Autodesk Fusion 360 part; units mm, degrees
(part 2 of 6)
  spline S50 degree 5 poles (26.1313, 46.3256) (26.12, 46.3173) (26.0976, 46.3005) (26.0639, 46.2753) (26.0191, 46.2416) (25.9633, 46.1993) (25.9077, 46.1569) (25.8522, 46.1143) (25.797, 46.0715) (25.7419, 46.0286) (25.687, 45.9856) (25.6324, 45.9424) (25.5779, 45.899) (25.5236, 45.8555) (25.4695, 45.8119) (25.4156, 45.768) (25.3619, 45.7241) (25.3084, 45.6799) (25.2552, 45.6356) (25.2021, 45.5912) (25.1492, 45.5466) (25.0966, 45.5018) (25.0441, 45.4569) (24.9919, 45.4118) (24.9399, 45.3665) (24.8881, 45.3211) (24.8365, 45.2755) (24.7851, 45.2297) (24.734, 45.1838) (24.6831, 45.1377) (24.6324, 45.0914) (24.582, 45.045) (24.5318, 44.9984) (24.4818, 44.9516) (24.4321, 44.9046) (24.3827, 44.8575) (24.3334, 44.8102) (24.2845, 44.7627) (24.2357, 44.7151) (24.1873, 44.6672) (24.1391, 44.6192) (24.0912, 44.571) (24.0435, 44.5226) (24.003, 44.481) (23.9721, 44.4491) (23.9507, 44.4268) (23.9388, 44.4144) (23.9362, 44.4117) knots -1 -1 -1 -1 -1 -1 -0.985714 -0.971429 -0.957143 -0.942857 -0.928571 -0.914286 -0.9 -0.885714 -0.871429 -0.857143 -0.842857 -0.828571 -0.814286 -0.8 -0.785714 -0.771429 -0.757143 -0.742857 -0.728571 -0.714286 -0.7 -0.685714 -0.671429 -0.657143 -0.642857 -0.628571 -0.614286 -0.6 -0.585714 -0.571429 -0.557143 -0.542857 -0.528571 -0.514286 -0.5 -0.485714 -0.471429 -0.457143 -0.442857 -0.428571 -0.414286 -0.4 -0.396066 -0.396066 -0.396066 -0.396066 -0.396066 -0.396066
  spline S51 degree 3 poles (23.3421, 44.3152) (23.3997, 44.2848) (23.4627, 44.266) (23.5923, 44.2536) (23.6577, 44.2602) (23.761, 44.2914) (23.8002, 44.309) (23.8731, 44.3538) (23.9066, 44.3808) (23.9362, 44.4117) knots 0 0 0 0 0.019532 0.019532 0.039064 0.039064 0.051902 0.051902 0.06474 0.06474 0.06474 0.06474
  arc A26 (23.3421, 44.3152) -> (22.9124, 44.5389) centre (0, 0) ccw
  spline S52 degree 3 poles (22.6507, 45.0809) (22.638, 45.017) (22.6379, 44.9513) (22.663, 44.8235) (22.6878, 44.7626) (22.7472, 44.6726) (22.7753, 44.64) (22.839, 44.5828) (22.8743, 44.5585) (22.9124, 44.5389) knots 0 0 0 0 0.019532 0.019532 0.039064 0.039064 0.051902 0.051902 0.06474 0.06474 0.06474 0.06474
  spline S53 degree 5 poles (22.6507, 45.0809) (22.6514, 45.0845) (22.6548, 45.1015) (22.6607, 45.1317) (22.6692, 45.1754) (22.68, 45.2324) (22.6923, 45.2992) (22.7043, 45.3661) (22.716, 45.4331) (22.7274, 45.5003) (22.7385, 45.5675) (22.7493, 45.6349) (22.7598, 45.7023) (22.77, 45.7699) (22.78, 45.8375) (22.7897, 45.9053) (22.799, 45.9731) (22.8081, 46.0411) (22.817, 46.1091) (22.8255, 46.1773) (22.8338, 46.2455) (22.8419, 46.3138) (22.8496, 46.3822) (22.8571, 46.4507) (22.8644, 46.5193) (22.8714, 46.5879) (22.8781, 46.6566) (22.8846, 46.7255) (22.8908, 46.7944) (22.8968, 46.8633) (22.9025, 46.9324) (22.908, 47.0015) (22.9132, 47.0707) (22.9182, 47.14) (22.9229, 47.2094) (22.9274, 47.2788) (22.9317, 47.3483) (22.9357, 47.4179) (22.9395, 47.4875) (22.9431, 47.5572) (22.9464, 47.627) (22.9495, 47.6968) (22.9523, 47.7667) (22.9549, 47.8367) (22.9569, 47.8927) (22.9582, 47.9347) (22.959, 47.9628) (22.9595, 47.9768) knots 0.396066 0.396066 0.396066 0.396066 0.396066 0.396066 0.4 0.414286 0.428571 0.442857 0.457143 0.471429 0.485714 0.5 0.514286 0.528571 0.542857 0.557143 0.571429 0.585714 0.6 0.614286 0.628571 0.642857 0.657143 0.671429 0.685714 0.7 0.714286 0.728571 0.742857 0.757143 0.771429 0.785714 0.8 0.814286 0.828571 0.842857 0.857143 0.871429 0.885714 0.9 0.914286 0.928571 0.942857 0.957143 0.971429 0.985714 1 1 1 1 1 1
  arc A27 (22.9595, 47.9768) -> (21.9943, 48.4269) centre (0, 0) ccw
  spline S54 degree 5 poles (21.9943, 48.4269) (21.9838, 48.4175) (21.9629, 48.3989) (21.9315, 48.3708) (21.8899, 48.3333) (21.8379, 48.2863) (21.7862, 48.2392) (21.7347, 48.192) (21.6834, 48.1446) (21.6323, 48.097) (21.5814, 48.0494) (21.5307, 48.0016) (21.4802, 47.9536) (21.4299, 47.9056) (21.3798, 47.8574) (21.33, 47.809) (21.2803, 47.7605) (21.2309, 47.7119) (21.1817, 47.6631) (21.1327, 47.6142) (21.0839, 47.5651) (21.0353, 47.5159) (20.987, 47.4666) (20.9389, 47.4171) (20.891, 47.3675) (20.8434, 47.3177) (20.796, 47.2678) (20.7488, 47.2178) (20.7019, 47.1676) (20.6552, 47.1172) (20.6087, 47.0667) (20.5625, 47.016) (20.5166, 46.9652) (20.4709, 46.9143) (20.4255, 46.8632) (20.3803, 46.8119) (20.3354, 46.7605) (20.2907, 46.7089) (20.2463, 46.6572) (20.2022, 46.6053) (20.1584, 46.5533) (20.1149, 46.501) (20.0716, 46.4487) (20.0349, 46.4038) (20.0069, 46.3692) (19.9875, 46.3452) (19.9767, 46.3318) (19.9744, 46.3288) knots -1 -1 -1 -1 -1 -1 -0.985714 -0.971429 -0.957143 -0.942857 -0.928571 -0.914286 -0.9 -0.885714 -0.871429 -0.857143 -0.842857 -0.828571 -0.814286 -0.8 -0.785714 -0.771429 -0.757143 -0.742857 -0.728571 -0.714286 -0.7 -0.685714 -0.671429 -0.657143 -0.642857 -0.628571 -0.614286 -0.6 -0.585714 -0.571429 -0.557143 -0.542857 -0.528571 -0.514286 -0.5 -0.485714 -0.471429 -0.457143 -0.442857 -0.428571 -0.414286 -0.4 -0.396066 -0.396066 -0.396066 -0.396066 -0.396066 -0.396066
  spline S55 degree 3 poles (19.391, 46.1809) (19.451, 46.1557) (19.5154, 46.1425) (19.6456, 46.1414) (19.7102, 46.1536) (19.8103, 46.1938) (19.8478, 46.2147) (19.9166, 46.2657) (19.9476, 46.2955) (19.9744, 46.3288) knots 0 0 0 0 0.019532 0.019532 0.039064 0.039064 0.051902 0.051902 0.06474 0.06474 0.06474 0.06474
  arc A28 (19.391, 46.1809) -> (18.9434, 46.3663) centre (0, 0) ccw
  spline S56 degree 3 poles (18.6354, 46.8834) (18.6284, 46.8187) (18.634, 46.7532) (18.6701, 46.6281) (18.7002, 46.5697) (18.7672, 46.4851) (18.798, 46.4551) (18.8664, 46.4037) (18.9038, 46.3825) (18.9434, 46.3663) knots 0 0 0 0 0.019532 0.019532 0.039064 0.039064 0.051902 0.051902 0.06474 0.06474 0.06474 0.06474
  spline S57 degree 5 poles (18.6354, 46.8834) (18.6358, 46.8872) (18.6377, 46.9043) (18.641, 46.935) (18.6456, 46.9792) (18.6514, 47.0369) (18.6578, 47.1046) (18.664, 47.1723) (18.6698, 47.2401) (18.6753, 47.3079) (18.6805, 47.3759) (18.6854, 47.4439) (18.69, 47.5121) (18.6943, 47.5802) (18.6983, 47.6485) (18.702, 47.7169) (18.7055, 47.7853) (18.7086, 47.8537) (18.7115, 47.9223) (18.7141, 47.9909) (18.7164, 48.0596) (18.7184, 48.1284) (18.7202, 48.1972) (18.7217, 48.2661) (18.723, 48.335) (18.7239, 48.404) (18.7246, 48.4731) (18.7251, 48.5422) (18.7253, 48.6114) (18.7252, 48.6806) (18.7249, 48.7499) (18.7243, 48.8192) (18.7235, 48.8886) (18.7224, 48.9581) (18.7211, 49.0276) (18.7196, 49.0971) (18.7177, 49.1667) (18.7157, 49.2364) (18.7134, 49.3061) (18.7109, 49.3758) (18.7081, 49.4456) (18.7051, 49.5155) (18.7018, 49.5854) (18.6984, 49.6553) (18.6954, 49.7113) (18.6931, 49.7533) (18.6914, 49.7813) (18.6906, 49.7953) knots 0.396066 0.396066 0.396066 0.396066 0.396066 0.396066 0.4 0.414286 0.428571 0.442857 0.457143 0.471429 0.485714 0.5 0.514286 0.528571 0.542857 0.557143 0.571429 0.585714 0.6 0.614286 0.628571 0.642857 0.657143 0.671429 0.685714 0.7 0.714286 0.728571 0.742857 0.757143 0.771429 0.785714 0.8 0.814286 0.828571 0.842857 0.857143 0.871429 0.885714 0.9 0.914286 0.928571 0.942857 0.957143 0.971429 0.985714 1 1 1 1 1 1
  arc A29 (18.6906, 49.7953) -> (17.6899, 50.1595) centre (0, 0) ccw
  spline S58 degree 5 poles (17.6899, 50.1595) (17.6803, 50.1493) (17.6611, 50.1289) (17.6323, 50.0982) (17.594, 50.0572) (17.5464, 50.0059) (17.499, 49.9544) (17.4518, 49.9029) (17.4048, 49.8512) (17.358, 49.7994) (17.3115, 49.7475) (17.2651, 49.6954) (17.219, 49.6433) (17.1731, 49.591) (17.1274, 49.5386) (17.082, 49.4861) (17.0367, 49.4335) (16.9917, 49.3807) (16.9469, 49.3278) (16.9024, 49.2748) (16.8581, 49.2217) (16.814, 49.1685) (16.7701, 49.1151) (16.7265, 49.0616) (16.6832, 49.008) (16.64, 48.9543) (16.5972, 48.9004) (16.5545, 48.8465) (16.5122, 48.7924) (16.47, 48.7381) (16.4282, 48.6838) (16.3866, 48.6293) (16.3452, 48.5747) (16.3041, 48.5199) (16.2633, 48.465) (16.2228, 48.41) (16.1825, 48.3549) (16.1426, 48.2996) (16.1029, 48.2442) (16.0634, 48.1887) (16.0243, 48.133) (15.9855, 48.0772) (15.947, 48.0213) (15.9143, 47.9733) (15.8894, 47.9365) (15.8722, 47.9109) (15.8626, 47.8965) (15.8605, 47.8934) knots -1 -1 -1 -1 -1 -1 -0.985714 -0.971429 -0.957143 -0.942857 -0.928571 -0.914286 -0.9 -0.885714 -0.871429 -0.857143 -0.842857 -0.828571 -0.814286 -0.8 -0.785714 -0.771429 -0.757143 -0.742857 -0.728571 -0.714286 -0.7 -0.685714 -0.671429 -0.657143 -0.642857 -0.628571 -0.614286 -0.6 -0.585714 -0.571429 -0.557143 -0.542857 -0.528571 -0.514286 -0.5 -0.485714 -0.471429 -0.457143 -0.442857 -0.428571 -0.414286 -0.4 -0.396066 -0.396066 -0.396066 -0.396066 -0.396066 -0.396066
  spline S59 degree 3 poles (15.2922, 47.6952) (15.3542, 47.6754) (15.4195, 47.6678) (15.5493, 47.6781) (15.6126, 47.6959) (15.7089, 47.7446) (15.7444, 47.7687) (15.8085, 47.8255) (15.8367, 47.8579) (15.8605, 47.8934) knots 0 0 0 0 0.019532 0.019532 0.039064 0.039064 0.051902 0.051902 0.06474 0.06474 0.06474 0.06474
  arc A30 (15.2922, 47.6952) -> (14.8302, 47.8409) centre (0, 0) ccw
  spline S60 degree 3 poles (14.4784, 48.3292) (14.477, 48.2641) (14.4883, 48.1994) (14.5351, 48.0779) (14.5702, 48.0223) (14.6443, 47.9439) (14.6776, 47.9167) (14.7502, 47.8715) (14.7893, 47.8536) (14.8302, 47.8409) knots 0 0 0 0 0.019532 0.019532 0.039064 0.039064 0.051902 0.051902 0.06474 0.06474 0.06474 0.06474
  spline S61 degree 5 poles (14.4784, 48.3292) (14.4784, 48.333) (14.4788, 48.3502) (14.4794, 48.3811) (14.4801, 48.4255) (14.4809, 48.4835) (14.4814, 48.5515) (14.4816, 48.6194) (14.4815, 48.6875) (14.4811, 48.7556) (14.4803, 48.8237) (14.4793, 48.8919) (14.4779, 48.9602) (14.4763, 49.0285) (14.4743, 49.0969) (14.4721, 49.1653) (14.4695, 49.2337) (14.4667, 49.3022) (14.4636, 49.3708) (14.4602, 49.4393) (14.4565, 49.508) (14.4525, 49.5766) (14.4483, 49.6453) (14.4438, 49.7141) (14.439, 49.7829) (14.434, 49.8517) (14.4287, 49.9206) (14.4231, 49.9895) (14.4173, 50.0584) (14.4112, 50.1274) (14.4048, 50.1964) (14.3982, 50.2654) (14.3913, 50.3345) (14.3842, 50.4035) (14.3768, 50.4727) (14.3692, 50.5418) (14.3614, 50.611) (14.3532, 50.6802) (14.3449, 50.7494) (14.3363, 50.8187) (14.3274, 50.888) (14.3183, 50.9573) (14.309, 51.0266) (14.2995, 51.096) (14.2916, 51.1515) (14.2856, 51.1931) (14.2816, 51.2209) (14.2796, 51.2348) knots 0.396066 0.396066 0.396066 0.396066 0.396066 0.396066 0.4 0.414286 0.428571 0.442857 0.457143 0.471429 0.485714 0.5 0.514286 0.528571 0.542857 0.557143 0.571429 0.585714 0.6 0.614286 0.628571 0.642857 0.657143 0.671429 0.685714 0.7 0.714286 0.728571 0.742857 0.757143 0.771429 0.785714 0.8 0.814286 0.828571 0.842857 0.857143 0.871429 0.885714 0.9 0.914286 0.928571 0.942857 0.957143 0.971429 0.985714 1 1 1 1 1 1
  arc A31 (14.2796, 51.2348) -> (13.2509, 51.5104) centre (0, 0) ccw
  spline S62 degree 5 poles (13.2509, 51.5104) (13.2422, 51.4994) (13.2248, 51.4774) (13.1988, 51.4443) (13.1643, 51.4002) (13.1213, 51.3449) (13.0786, 51.2895) (13.0361, 51.234) (12.9938, 51.1784) (12.9517, 51.1228) (12.9098, 51.067) (12.8682, 51.0111) (12.8268, 50.9551) (12.7856, 50.899) (12.7447, 50.8429) (12.704, 50.7866) (12.6635, 50.7302) (12.6232, 50.6737) (12.5832, 50.6172) (12.5435, 50.5605) (12.504, 50.5037) (12.4647, 50.4468) (12.4257, 50.3898) (12.3869, 50.3328) (12.3483, 50.2756) (12.3101, 50.2183) (12.272, 50.1609) (12.2343, 50.1034) (12.1968, 50.0458) (12.1596, 49.9881) (12.1226, 49.9303) (12.0859, 49.8724) (12.0495, 49.8144) (12.0133, 49.7563) (11.9774, 49.6981) (11.9419, 49.6397) (11.9065, 49.5813) (11.8715, 49.5228) (11.8368, 49.4641) (11.8024, 49.4053) (11.7683, 49.3465) (11.7345, 49.2875) (11.701, 49.2284) (11.6726, 49.1778) (11.651, 49.139) (11.6361, 49.1119) (11.6278, 49.0968) (11.626, 49.0935) knots -1 -1 -1 -1 -1 -1 -0.985714 -0.971429 -0.957143 -0.942857 -0.928571 -0.914286 -0.9 -0.885714 -0.871429 -0.857143 -0.842857 -0.828571 -0.814286 -0.8 -0.785714 -0.771429 -0.757143 -0.742857 -0.728571 -0.714286 -0.7 -0.685714 -0.671429 -0.657143 -0.642857 -0.628571 -0.614286 -0.6 -0.585714 -0.571429 -0.557143 -0.542857 -0.528571 -0.514286 -0.5 -0.485714 -0.471429 -0.457143 -0.442857 -0.428571 -0.414286 -0.4 -0.396066 -0.396066 -0.396066 -0.396066 -0.396066 -0.396066
  spline S63 degree 3 poles (11.0771, 48.8466) (11.1406, 48.8322) (11.2063, 48.8303) (11.3347, 48.8519) (11.3962, 48.8751) (11.4879, 48.932) (11.5212, 48.9592) (11.5801, 49.0213) (11.6054, 49.056) (11.626, 49.0935) knots 0 0 0 0 0.019532 0.019532 0.039064 0.039064 0.051902 0.051902 0.06474 0.06474 0.06474 0.06474
  arc A32 (11.0771, 48.8466) -> (10.6042, 48.9514) centre (0, 0) ccw
  spline S64 degree 3 poles (10.2111, 49.4072) (10.2154, 49.3422) (10.2323, 49.2787) (10.2896, 49.1618) (10.3293, 49.1094) (10.41, 49.0378) (10.4455, 49.0136) (10.5218, 48.9749) (10.5623, 48.9605) (10.6042, 48.9514) knots 0 0 0 0 0.019532 0.019532 0.039064 0.039064 0.051902 0.051902 0.06474 0.06474 0.06474 0.06474
  spline S65 degree 5 poles (10.2111, 49.4072) (10.2109, 49.4109) (10.2097, 49.4282) (10.2076, 49.4589) (10.2045, 49.5033) (10.2002, 49.5611) (10.1948, 49.6288) (10.189, 49.6966) (10.183, 49.7644) (10.1766, 49.8322) (10.17, 49.9) (10.163, 49.9678) (10.1557, 50.0357) (10.1481, 50.1036) (10.1402, 50.1715) (10.132, 50.2395) (10.1235, 50.3075) (10.1147, 50.3755) (10.1056, 50.4435) (10.0962, 50.5115) (10.0866, 50.5795) (10.0767, 50.6476) (10.0665, 50.7157) (10.056, 50.7838) (10.0452, 50.8519) (10.0342, 50.92) (10.0229, 50.9881) (10.0114, 51.0563) (9.9995, 51.1245) (9.9874, 51.1926) (9.9751, 51.2608) (9.9625, 51.329) (9.9496, 51.3972) (9.9365, 51.4654) (9.9232, 51.5336) (9.9095, 51.6019) (9.8957, 51.6701) (9.8816, 51.7383) (9.8672, 51.8066) (9.8526, 51.8748) (9.8377, 51.9431) (9.8226, 52.0113) (9.8073, 52.0796) (9.7917, 52.1478) (9.7791, 52.2025) (9.7695, 52.2434) (9.7631, 52.2707) (9.7598, 52.2844) knots 0.396066 0.396066 0.396066 0.396066 0.396066 0.396066 0.4 0.414286 0.428571 0.442857 0.457143 0.471429 0.485714 0.5 0.514286 0.528571 0.542857 0.557143 0.571429 0.585714 0.6 0.614286 0.628571 0.642857 0.657143 0.671429 0.685714 0.7 0.714286 0.728571 0.742857 0.757143 0.771429 0.785714 0.8 0.814286 0.828571 0.842857 0.857143 0.871429 0.885714 0.9 0.914286 0.928571 0.942857 0.957143 0.971429 0.985714 1 1 1 1 1 1
  arc A33 (9.7598, 52.2844) -> (8.7111, 52.4693) centre (0, 0) ccw
  spline S66 degree 5 poles (8.7111, 52.4693) (8.7034, 52.4576) (8.688, 52.4341) (8.665, 52.3989) (8.6344, 52.3519) (8.5964, 52.2931) (8.5587, 52.2342) (8.5211, 52.1752) (8.4838, 52.1162) (8.4468, 52.057) (8.4099, 51.9978) (8.3733, 51.9385) (8.337, 51.8791) (8.3008, 51.8197) (8.2649, 51.7602) (8.2293, 51.7006) (8.1939, 51.6409) (8.1587, 51.5811) (8.1238, 51.5212) (8.0891, 51.4613) (8.0547, 51.4013) (8.0205, 51.3412) (7.9866, 51.2811) (7.9529, 51.2208) (7.9196, 51.1605) (7.8864, 51.1001) (7.8535, 51.0396) (7.8209, 50.979) (7.7886, 50.9184) (7.7565, 50.8577) (7.7247, 50.7969) (7.6932, 50.736) (7.662, 50.675) (7.6311, 50.614) (7.6004, 50.5528) (7.57, 50.4916) (7.5399, 50.4303) (7.5102, 50.369) (7.4807, 50.3075) (7.4515, 50.246) (7.4227, 50.1844) (7.3941, 50.1227) (7.3659, 50.0609) (7.342, 50.008) (7.3239, 49.9674) (7.3114, 49.9392) (7.3045, 49.9234) (7.303, 49.92) knots -1 -1 -1 -1 -1 -1 -0.985714 -0.971429 -0.957143 -0.942857 -0.928571 -0.914286 -0.9 -0.885714 -0.871429 -0.857143 -0.842857 -0.828571 -0.814286 -0.8 -0.785714 -0.771429 -0.757143 -0.742857 -0.728571 -0.714286 -0.7 -0.685714 -0.671429 -0.657143 -0.642857 -0.628571 -0.614286 -0.6 -0.585714 -0.571429 -0.557143 -0.542857 -0.528571 -0.514286 -0.5 -0.485714 -0.471429 -0.457143 -0.442857 -0.428571 -0.414286 -0.4 -0.396066 -0.396066 -0.396066 -0.396066 -0.396066 -0.396066
  spline S67 degree 3 poles (6.7777, 49.6261) (6.8422, 49.6173) (6.9078, 49.6212) (7.0339, 49.6539) (7.0931, 49.6824) (7.1795, 49.7471) (7.2103, 49.777) (7.2635, 49.844) (7.2857, 49.8808) (7.303, 49.92) knots 0 0 0 0 0.019532 0.019532 0.039064 0.039064 0.051902 0.051902 0.06474 0.06474 0.06474 0.06474
  arc A34 (6.7777, 49.6261) -> (6.2974, 49.6893) centre (0, 0) ccw
  spline S68 degree 3 poles (5.8661, 50.1091) (5.876, 50.0448) (5.8984, 49.983) (5.9657, 49.8715) (6.0099, 49.8228) (6.0965, 49.7585) (6.134, 49.7375) (6.2134, 49.7055) (6.255, 49.6947) (6.2974, 49.6893) knots 0 0 0 0 0.019532 0.019532 0.039064 0.039064 0.051902 0.051902 0.06474 0.06474 0.06474 0.06474
  spline S69 degree 5 poles (5.8661, 50.1091) (5.8656, 50.1128) (5.8629, 50.1299) (5.8581, 50.1604) (5.8512, 50.2043) (5.8418, 50.2615) (5.8305, 50.3285) (5.8189, 50.3955) (5.807, 50.4625) (5.7947, 50.5295) (5.7822, 50.5965) (5.7693, 50.6635) (5.7561, 50.7304) (5.7426, 50.7974) (5.7288, 50.8644) (5.7147, 50.9314) (5.7003, 50.9984) (5.6857, 51.0653) (5.6707, 51.1323) (5.6554, 51.1992) (5.6399, 51.2662) (5.6241, 51.3331) (5.608, 51.4) (5.5916, 51.467) (5.575, 51.5339) (5.558, 51.6008) (5.5409, 51.6677) (5.5234, 51.7346) (5.5057, 51.8014) (5.4877, 51.8683) (5.4695, 51.9351) (5.451, 52.002) (5.4322, 52.0688) (5.4132, 52.1356) (5.3939, 52.2024) (5.3744, 52.2692) (5.3547, 52.3359) (5.3347, 52.4027) (5.3144, 52.4694) (5.2939, 52.5361) (5.2732, 52.6028) (5.2522, 52.6695) (5.231, 52.7362) (5.2095, 52.8028) (5.1921, 52.8561) (5.179, 52.8961) (5.1702, 52.9227) (5.1658, 52.936) knots 0.396066 0.396066 0.396066 0.396066 0.396066 0.396066 0.4 0.414286 0.428571 0.442857 0.457143 0.471429 0.485714 0.5 0.514286 0.528571 0.542857 0.557143 0.571429 0.585714 0.6 0.614286 0.628571 0.642857 0.657143 0.671429 0.685714 0.7 0.714286 0.728571 0.742857 0.757143 0.771429 0.785714 0.8 0.814286 0.828571 0.842857 0.857143 0.871429 0.885714 0.9 0.914286 0.928571 0.942857 0.957143 0.971429 0.985714 1 1 1 1 1 1
  arc A35 (5.1658, 52.936) -> (4.1049, 53.0289) centre (0, 0) ccw
  spline S70 degree 5 poles (4.1049, 53.0289) (4.0983, 53.0165) (4.085, 52.9918) (4.0651, 52.9547) (4.0388, 52.9052) (4.0061, 52.8433) (3.9736, 52.7814) (3.9413, 52.7193) (3.9093, 52.6573) (3.8776, 52.5951) (3.846, 52.5329) (3.8147, 52.4707) (3.7837, 52.4083) (3.7529, 52.346) (3.7223, 52.2835) (3.692, 52.221) (3.6619, 52.1585) (3.6321, 52.0959) (3.6025, 52.0332) (3.5732, 51.9705) (3.5441, 51.9077) (3.5153, 51.8449) (3.4868, 51.782) (3.4585, 51.719) (3.4305, 51.656) (3.4027, 51.593) (3.3753, 51.5299) (3.3481, 51.4667) (3.3211, 51.4035) (3.2945, 51.3402) (3.2681, 51.2768) (3.242, 51.2134) (3.2162, 51.15) (3.1907, 51.0865) (3.1655, 51.0229) (3.1406, 50.9593) (3.116, 50.8956) (3.0916, 50.8319) (3.0676, 50.7681) (3.0439, 50.7042) (3.0206, 50.6403) (2.9975, 50.5764) (2.9748, 50.5124) (2.9556, 50.4576) (2.9411, 50.4156) (2.9311, 50.3864) (2.9256, 50.37) (2.9244, 50.3665) knots -1 -1 -1 -1 -1 -1 -0.985714 -0.971429 -0.957143 -0.942857 -0.928571 -0.914286 -0.9 -0.885714 -0.871429 -0.857143 -0.842857 -0.828571 -0.814286 -0.8 -0.785714 -0.771429 -0.757143 -0.742857 -0.728571 -0.714286 -0.7 -0.685714 -0.671429 -0.657143 -0.642857 -0.628571 -0.614286 -0.6 -0.585714 -0.571429 -0.557143 -0.542857 -0.528571 -0.514286 -0.5 -0.485714 -0.471429 -0.457143 -0.442857 -0.428571 -0.414286 -0.4 -0.396066 -0.396066 -0.396066 -0.396066 -0.396066 -0.396066
  spline S71 degree 3 poles (2.4267, 50.028) (2.4918, 50.0248) (2.5568, 50.0344) (2.6795, 50.078) (2.736, 50.1115) (2.8164, 50.1835) (2.8445, 50.216) (2.8917, 50.2874) (2.9106, 50.326) (2.9244, 50.3665) knots 0 0 0 0 0.019532 0.019532 0.039064 0.039064 0.051902 0.051902 0.06474 0.06474 0.06474 0.06474
  arc A36 (2.4267, 50.028) -> (1.9427, 50.0491) centre (0, 0) ccw
  spline S72 degree 3 poles (1.4765, 50.4297) (1.492, 50.3665) (1.5197, 50.3069) (1.5964, 50.2017) (1.6446, 50.157) (1.7365, 50.1005) (1.7757, 50.0828) (1.8576, 50.0579) (1.9, 50.0508) (1.9427, 50.0491) knots 0 0 0 0 0.019532 0.019532 0.039064 0.039064 0.051902 0.051902 0.06474 0.06474 0.06474 0.06474
  spline S73 degree 5 poles (1.4765, 50.4297) (1.4756, 50.4334) (1.4715, 50.4501) (1.4641, 50.4801) (1.4533, 50.5232) (1.439, 50.5794) (1.4219, 50.6452) (1.4045, 50.7109) (1.3868, 50.7766) (1.3688, 50.8423) (1.3504, 50.9079) (1.3317, 50.9735) (1.3128, 51.0391) (1.2935, 51.1046) (1.2739, 51.1702) (1.254, 51.2356) (1.2339, 51.3011) (1.2134, 51.3665) (1.1926, 51.4319) (1.1716, 51.4973) (1.1503, 51.5626) (1.1287, 51.6279) (1.1068, 51.6932) (1.0847, 51.7585) (1.0623, 51.8237) (1.0396, 51.8888) (1.0166, 51.954) (0.9934, 52.0191) (0.9699, 52.0842) (0.9462, 52.1492) (0.9222, 52.2142) (0.898, 52.2792) (0.8734, 52.3441) (0.8487, 52.409) (0.8237, 52.4739) (0.7984, 52.5387) (0.7729, 52.6035) (0.7472, 52.6682) (0.7212, 52.7329) (0.6949, 52.7976) (0.6685, 52.8622) (0.6417, 52.9268) (0.6148, 52.9914) (0.5876, 53.0559) (0.5657, 53.1075) (0.5491, 53.1462) (0.538, 53.1719) (0.5325, 53.1848) knots 0.396066 0.396066 0.396066 0.396066 0.396066 0.396066 0.4 0.414286 0.428571 0.442857 0.457143 0.471429 0.485714 0.5 0.514286 0.528571 0.542857 0.557143 0.571429 0.585714 0.6 0.614286 0.628571 0.642857 0.657143 0.671429 0.685714 0.7 0.714286 0.728571 0.742857 0.757143 0.771429 0.785714 0.8 0.814286 0.828571 0.842857 0.857143 0.871429 0.885714 0.9 0.914286 0.928571 0.942857 0.957143 0.971429 0.985714 1 1 1 1 1 1
  arc A37 (0.5325, 53.1848) -> (-0.5325, 53.1848) centre (0, 0) ccw
  spline S74 degree 5 poles (-0.5325, 53.1848) (-0.538, 53.1719) (-0.5491, 53.1462) (-0.5657, 53.1075) (-0.5876, 53.0559) (-0.6148, 52.9914) (-0.6417, 52.9268) (-0.6685, 52.8622) (-0.6949, 52.7976) (-0.7212, 52.7329) (-0.7472, 52.6682) (-0.7729, 52.6035) (-0.7984, 52.5387) (-0.8237, 52.4739) (-0.8487, 52.409) (-0.8734, 52.3441) (-0.898, 52.2792) (-0.9222, 52.2142) (-0.9462, 52.1492) (-0.9699, 52.0842) (-0.9934, 52.0191) (-1.0166, 51.954) (-1.0396, 51.8888) (-1.0623, 51.8237) (-1.0847, 51.7585) (-1.1068, 51.6932) (-1.1287, 51.6279) (-1.1503, 51.5626) (-1.1716, 51.4973) (-1.1926, 51.4319) (-1.2134, 51.3665) (-1.2339, 51.3011) (-1.254, 51.2356) (-1.2739, 51.1702) (-1.2935, 51.1046) (-1.3128, 51.0391) (-1.3317, 50.9735) (-1.3504, 50.9079) (-1.3688, 50.8423) (-1.3868, 50.7766) (-1.4045, 50.7109) (-1.4219, 50.6452) (-1.439, 50.5794) (-1.4533, 50.5232) (-1.4641, 50.4801) (-1.4715, 50.4501) (-1.4756, 50.4334) (-1.4765, 50.4297) knots -1 -1 -1 -1 -1 -1 -0.985714 -0.971429 -0.957143 -0.942857 -0.928571 -0.914286 -0.9 -0.885714 -0.871429 -0.857143 -0.842857 -0.828571 -0.814286 -0.8 -0.785714 -0.771429 -0.757143 -0.742857 -0.728571 -0.714286 -0.7 -0.685714 -0.671429 -0.657143 -0.642857 -0.628571 -0.614286 -0.6 -0.585714 -0.571429 -0.557143 -0.542857 -0.528571 -0.514286 -0.5 -0.485714 -0.471429 -0.457143 -0.442857 -0.428571 -0.414286 -0.4 -0.396066 -0.396066 -0.396066 -0.396066 -0.396066 -0.396066
  spline S75 degree 3 poles (-1.9427, 50.0491) (-1.8777, 50.0516) (-1.8137, 50.0669) (-1.6953, 50.1209) (-1.6419, 50.1593) (-1.5681, 50.238) (-1.543, 50.2728) (-1.5022, 50.3481) (-1.4867, 50.3882) (-1.4765, 50.4297) knots 0 0 0 0 0.019532 0.019532 0.039064 0.039064 0.051902 0.051902 0.06474 0.06474 0.06474 0.06474
  arc A38 (-1.9427, 50.0491) -> (-2.4267, 50.028) centre (0, 0) ccw
  spline S76 degree 3 poles (-2.9244, 50.3665) (-2.9034, 50.3049) (-2.8706, 50.2479) (-2.785, 50.1498) (-2.7331, 50.1095) (-2.6366, 50.0612) (-2.596, 50.047) (-2.5123, 50.0293) (-2.4695, 50.0259) (-2.4267, 50.028) knots 0 0 0 0 0.019532 0.019532 0.039064 0.039064 0.051902 0.051902 0.06474 0.06474 0.06474 0.06474
  spline S77 degree 5 poles (-2.9244, 50.3665) (-2.9256, 50.37) (-2.9311, 50.3864) (-2.9411, 50.4156) (-2.9556, 50.4576) (-2.9748, 50.5124) (-2.9975, 50.5764) (-3.0206, 50.6403) (-3.0439, 50.7042) (-3.0676, 50.7681) (-3.0916, 50.8319) (-3.116, 50.8956) (-3.1406, 50.9593) (-3.1655, 51.0229) (-3.1907, 51.0865) (-3.2162, 51.15) (-3.242, 51.2134) (-3.2681, 51.2768) (-3.2945, 51.3402) (-3.3211, 51.4035) (-3.3481, 51.4667) (-3.3753, 51.5299) (-3.4027, 51.593) (-3.4305, 51.656) (-3.4585, 51.719) (-3.4868, 51.782) (-3.5153, 51.8449) (-3.5441, 51.9077) (-3.5732, 51.9705) (-3.6025, 52.0332) (-3.6321, 52.0959) (-3.6619, 52.1585) (-3.692, 52.221) (-3.7223, 52.2835) (-3.7529, 52.346) (-3.7837, 52.4083) (-3.8147, 52.4707) (-3.846, 52.5329) (-3.8776, 52.5951) (-3.9093, 52.6573) (-3.9413, 52.7193) (-3.9736, 52.7814) (-4.0061, 52.8433) (-4.0388, 52.9052) (-4.0651, 52.9547) (-4.085, 52.9918) (-4.0983, 53.0165) (-4.1049, 53.0289) knots 0.396066 0.396066 0.396066 0.396066 0.396066 0.396066 0.4 0.414286 0.428571 0.442857 0.457143 0.471429 0.485714 0.5 0.514286 0.528571 0.542857 0.557143 0.571429 0.585714 0.6 0.614286 0.628571 0.642857 0.657143 0.671429 0.685714 0.7 0.714286 0.728571 0.742857 0.757143 0.771429 0.785714 0.8 0.814286 0.828571 0.842857 0.857143 0.871429 0.885714 0.9 0.914286 0.928571 0.942857 0.957143 0.971429 0.985714 1 1 1 1 1 1
  arc A39 (-4.1049, 53.0289) -> (-5.1658, 52.936) centre (0, 0) ccw
  spline S78 degree 5 poles (-5.1658, 52.936) (-5.1702, 52.9227) (-5.179, 52.8961) (-5.1921, 52.8561) (-5.2095, 52.8028) (-5.231, 52.7362) (-5.2522, 52.6695) (-5.2732, 52.6028) (-5.2939, 52.5361) (-5.3144, 52.4694) (-5.3347, 52.4027) (-5.3547, 52.3359) (-5.3744, 52.2692) (-5.3939, 52.2024) (-5.4132, 52.1356) (-5.4322, 52.0688) (-5.451, 52.002) (-5.4695, 51.9351) (-5.4877, 51.8683) (-5.5057, 51.8014) (-5.5234, 51.7346) (-5.5409, 51.6677) (-5.558, 51.6008) (-5.575, 51.5339) (-5.5916, 51.467) (-5.608, 51.4) (-5.6241, 51.3331) (-5.6399, 51.2662) (-5.6554, 51.1992) (-5.6707, 51.1323) (-5.6857, 51.0653) (-5.7003, 50.9984) (-5.7147, 50.9314) (-5.7288, 50.8644) (-5.7426, 50.7974) (-5.7561, 50.7304) (-5.7693, 50.6635) (-5.7822, 50.5965) (-5.7947, 50.5295) (-5.807, 50.4625) (-5.8189, 50.3955) (-5.8305, 50.3285) (-5.8418, 50.2615) (-5.8512, 50.2043) (-5.8581, 50.1604) (-5.8629, 50.1299) (-5.8656, 50.1128) (-5.8661, 50.1091) knots -1 -1 -1 -1 -1 -1 -0.985714 -0.971429 -0.957143 -0.942857 -0.928571 -0.914286 -0.9 -0.885714 -0.871429 -0.857143 -0.842857 -0.828571 -0.814286 -0.8 -0.785714 -0.771429 -0.757143 -0.742857 -0.728571 -0.714286 -0.7 -0.685714 -0.671429 -0.657143 -0.642857 -0.628571 -0.614286 -0.6 -0.585714 -0.571429 -0.557143 -0.542857 -0.528571 -0.514286 -0.5 -0.485714 -0.471429 -0.457143 -0.442857 -0.428571 -0.414286 -0.4 -0.396066 -0.396066 -0.396066 -0.396066 -0.396066 -0.396066
  spline S79 degree 3 poles (-6.2974, 49.6893) (-6.2328, 49.6975) (-6.1704, 49.7183) (-6.0571, 49.7824) (-6.0073, 49.8253) (-5.9407, 49.9102) (-5.9186, 49.9471) (-5.8846, 50.0256) (-5.8726, 50.0668) (-5.8661, 50.1091) knots 0 0 0 0 0.019532 0.019532 0.039064 0.039064 0.051902 0.051902 0.06474 0.06474 0.06474 0.06474
  arc A40 (-6.2974, 49.6893) -> (-6.7777, 49.6261) centre (0, 0) ccw
  spline S80 degree 3 poles (-7.303, 49.92) (-7.2767, 49.8604) (-7.2391, 49.8065) (-7.1453, 49.7162) (-7.09, 49.6806) (-6.9897, 49.6409) (-6.9481, 49.6303) (-6.8631, 49.62) (-6.8201, 49.6203) (-6.7777, 49.6261) knots 0 0 0 0 0.019532 0.019532 0.039064 0.039064 0.051902 0.051902 0.06474 0.06474 0.06474 0.06474
  spline S81 degree 5 poles (-7.303, 49.92) (-7.3045, 49.9234) (-7.3114, 49.9392) (-7.3239, 49.9674) (-7.342, 50.008) (-7.3659, 50.0609) (-7.3941, 50.1227) (-7.4227, 50.1844) (-7.4515, 50.246) (-7.4807, 50.3075) (-7.5102, 50.369) (-7.5399, 50.4303) (-7.57, 50.4916) (-7.6004, 50.5528) (-7.6311, 50.614) (-7.662, 50.675) (-7.6932, 50.736) (-7.7247, 50.7969) (-7.7565, 50.8577) (-7.7886, 50.9184) (-7.8209, 50.979) (-7.8535, 51.0396) (-7.8864, 51.1001) (-7.9196, 51.1605) (-7.9529, 51.2208) (-7.9866, 51.2811) (-8.0205, 51.3412) (-8.0547, 51.4013) (-8.0891, 51.4613) (-8.1238, 51.5212) (-8.1587, 51.5811) (-8.1939, 51.6409) (-8.2293, 51.7006) (-8.2649, 51.7602) (-8.3008, 51.8197) (-8.337, 51.8791) (-8.3733, 51.9385) (-8.4099, 51.9978) (-8.4468, 52.057) (-8.4838, 52.1162) (-8.5211, 52.1752) (-8.5587, 52.2342) (-8.5964, 52.2931) (-8.6344, 52.3519) (-8.665, 52.3989) (-8.688, 52.4341) (-8.7034, 52.4576) (-8.7111, 52.4693) knots 0.396066 0.396066 0.396066 0.396066 0.396066 0.396066 0.4 0.414286 0.428571 0.442857 0.457143 0.471429 0.485714 0.5 0.514286 0.528571 0.542857 0.557143 0.571429 0.585714 0.6 0.614286 0.628571 0.642857 0.657143 0.671429 0.685714 0.7 0.714286 0.728571 0.742857 0.757143 0.771429 0.785714 0.8 0.814286 0.828571 0.842857 0.857143 0.871429 0.885714 0.9 0.914286 0.928571 0.942857 0.957143 0.971429 0.985714 1 1 1 1 1 1
  arc A41 (-8.7111, 52.4693) -> (-9.7598, 52.2844) centre (0, 0) ccw
  spline S82 degree 5 poles (-9.7598, 52.2844) (-9.7631, 52.2707) (-9.7695, 52.2434) (-9.7791, 52.2025) (-9.7917, 52.1478) (-9.8073, 52.0796) (-9.8226, 52.0113) (-9.8377, 51.9431) (-9.8526, 51.8748) (-9.8672, 51.8066) (-9.8816, 51.7383) (-9.8957, 51.6701) (-9.9095, 51.6019) (-9.9232, 51.5336) (-9.9365, 51.4654) (-9.9496, 51.3972) (-9.9625, 51.329) (-9.9751, 51.2608) (-9.9874, 51.1926) (-9.9995, 51.1245) (-10.0114, 51.0563) (-10.0229, 50.9881) (-10.0342, 50.92) (-10.0452, 50.8519) (-10.056, 50.7838) (-10.0665, 50.7157) (-10.0767, 50.6476) (-10.0866, 50.5795) (-10.0962, 50.5115) (-10.1056, 50.4435) (-10.1147, 50.3755) (-10.1235, 50.3075) (-10.132, 50.2395) (-10.1402, 50.1715) (-10.1481, 50.1036) (-10.1557, 50.0357) (-10.163, 49.9678) (-10.17, 49.9) (-10.1766, 49.8322) (-10.183, 49.7644) (-10.189, 49.6966) (-10.1948, 49.6288) (-10.2002, 49.5611) (-10.2045, 49.5033) (-10.2076, 49.4589) (-10.2097, 49.4282) (-10.2109, 49.4109) (-10.2111, 49.4072) knots -1 -1 -1 -1 -1 -1 -0.985714 -0.971429 -0.957143 -0.942857 -0.928571 -0.914286 -0.9 -0.885714 -0.871429 -0.857143 -0.842857 -0.828571 -0.814286 -0.8 -0.785714 -0.771429 -0.757143 -0.742857 -0.728571 -0.714286 -0.7 -0.685714 -0.671429 -0.657143 -0.642857 -0.628571 -0.614286 -0.6 -0.585714 -0.571429 -0.557143 -0.542857 -0.528571 -0.514286 -0.5 -0.485714 -0.471429 -0.457143 -0.442857 -0.428571 -0.414286 -0.4 -0.396066 -0.396066 -0.396066 -0.396066 -0.396066 -0.396066
  spline S83 degree 3 poles (-10.6042, 48.9514) (-10.5405, 48.9652) (-10.4802, 48.9913) (-10.3729, 49.0651) (-10.327, 49.1121) (-10.268, 49.2025) (-10.2493, 49.2411) (-10.2222, 49.3223) (-10.2139, 49.3645) (-10.2111, 49.4072) knots 0 0 0 0 0.019532 0.019532 0.039064 0.039064 0.051902 0.051902 0.06474 0.06474 0.06474 0.06474
  arc A42 (-10.6042, 48.9514) -> (-11.0771, 48.8466) centre (0, 0) ccw
  spline S84 degree 3 poles (-11.626, 49.0935) (-11.5946, 49.0365) (-11.5525, 48.986) (-11.4512, 48.9042) (-11.393, 48.8736) (-11.2896, 48.8428) (-11.2472, 48.8359) (-11.1616, 48.833) (-11.1189, 48.8371) (-11.0771, 48.8466) knots 0 0 0 0 0.019532 0.019532 0.039064 0.039064 0.051902 0.051902 0.06474 0.06474 0.06474 0.06474
  spline S85 degree 5 poles (-11.626, 49.0935) (-11.6278, 49.0968) (-11.6361, 49.1119) (-11.651, 49.139) (-11.6726, 49.1778) (-11.701, 49.2284) (-11.7345, 49.2875) (-11.7683, 49.3465) (-11.8024, 49.4053) (-11.8368, 49.4641) (-11.8715, 49.5228) (-11.9065, 49.5813) (-11.9419, 49.6397) (-11.9774, 49.6981) (-12.0133, 49.7563) (-12.0495, 49.8144) (-12.0859, 49.8724) (-12.1226, 49.9303) (-12.1596, 49.9881) (-12.1968, 50.0458) (-12.2343, 50.1034) (-12.272, 50.1609) (-12.3101, 50.2183) (-12.3483, 50.2756) (-12.3869, 50.3328) (-12.4257, 50.3898) (-12.4647, 50.4468) (-12.504, 50.5037) (-12.5435, 50.5605) (-12.5832, 50.6172) (-12.6232, 50.6737) (-12.6635, 50.7302) (-12.704, 50.7866) (-12.7447, 50.8429) (-12.7856, 50.899) (-12.8268, 50.9551) (-12.8682, 51.0111) (-12.9098, 51.067) (-12.9517, 51.1228) (-12.9938, 51.1784) (-13.0361, 51.234) (-13.0786, 51.2895) (-13.1213, 51.3449) (-13.1643, 51.4002) (-13.1988, 51.4443) (-13.2248, 51.4774) (-13.2422, 51.4994) (-13.2509, 51.5104) knots 0.396066 0.396066 0.396066 0.396066 0.396066 0.396066 0.4 0.414286 0.428571 0.442857 0.457143 0.471429 0.485714 0.5 0.514286 0.528571 0.542857 0.557143 0.571429 0.585714 0.6 0.614286 0.628571 0.642857 0.657143 0.671429 0.685714 0.7 0.714286 0.728571 0.742857 0.757143 0.771429 0.785714 0.8 0.814286 0.828571 0.842857 0.857143 0.871429 0.885714 0.9 0.914286 0.928571 0.942857 0.957143 0.971429 0.985714 1 1 1 1 1 1
  arc A43 (-13.2509, 51.5104) -> (-14.2796, 51.2348) centre (0, 0) ccw
  spline S86 degree 5 poles (-14.2796, 51.2348) (-14.2816, 51.2209) (-14.2856, 51.1931) (-14.2916, 51.1515) (-14.2995, 51.096) (-14.309, 51.0266) (-14.3183, 50.9573) (-14.3274, 50.888) (-14.3363, 50.8187) (-14.3449, 50.7494) (-14.3532, 50.6802) (-14.3614, 50.611) (-14.3692, 50.5418) (-14.3768, 50.4727) (-14.3842, 50.4035) (-14.3913, 50.3345) (-14.3982, 50.2654) (-14.4048, 50.1964) (-14.4112, 50.1274) (-14.4173, 50.0584) (-14.4231, 49.9895) (-14.4287, 49.9206) (-14.434, 49.8517) (-14.439, 49.7829) (-14.4438, 49.7141) (-14.4483, 49.6453) (-14.4525, 49.5766) (-14.4565, 49.508) (-14.4602, 49.4393) (-14.4636, 49.3708) (-14.4667, 49.3022) (-14.4695, 49.2337) (-14.4721, 49.1653) (-14.4743, 49.0969) (-14.4763, 49.0285) (-14.4779, 48.9602) (-14.4793, 48.8919) (-14.4803, 48.8237) (-14.4811, 48.7556) (-14.4815, 48.6875) (-14.4816, 48.6194) (-14.4814, 48.5515) (-14.4809, 48.4835) (-14.4801, 48.4255) (-14.4794, 48.3811) (-14.4788, 48.3502) (-14.4784, 48.333) (-14.4784, 48.3292) knots -1 -1 -1 -1 -1 -1 -0.985714 -0.971429 -0.957143 -0.942857 -0.928571 -0.914286 -0.9 -0.885714 -0.871429 -0.857143 -0.842857 -0.828571 -0.814286 -0.8 -0.785714 -0.771429 -0.757143 -0.742857 -0.728571 -0.714286 -0.7 -0.685714 -0.671429 -0.657143 -0.642857 -0.628571 -0.614286 -0.6 -0.585714 -0.571429 -0.557143 -0.542857 -0.528571 -0.514286 -0.5 -0.485714 -0.471429 -0.457143 -0.442857 -0.428571 -0.414286 -0.4 -0.396066 -0.396066 -0.396066 -0.396066 -0.396066 -0.396066
  spline S87 degree 3 poles (-14.8302, 47.8409) (-14.768, 47.8602) (-14.7102, 47.8914) (-14.6098, 47.9743) (-14.5681, 48.0252) (-14.5172, 48.1203) (-14.5019, 48.1605) (-14.482, 48.2437) (-14.4774, 48.2864) (-14.4784, 48.3292) knots 0 0 0 0 0.019532 0.019532 0.039064 0.039064 0.051902 0.051902 0.06474 0.06474 0.06474 0.06474
  arc A44 (-14.8302, 47.8409) -> (-15.2922, 47.6952) centre (0, 0) ccw
  spline S88 degree 3 poles (-15.8605, 47.8934) (-15.8243, 47.8393) (-15.7779, 47.7928) (-15.6699, 47.7201) (-15.6093, 47.6947) (-15.5036, 47.673) (-15.4607, 47.6698) (-15.3752, 47.6744) (-15.333, 47.6822) (-15.2922, 47.6952) knots 0 0 0 0 0.019532 0.019532 0.039064 0.039064 0.051902 0.051902 0.06474 0.06474 0.06474 0.06474
  spline S89 degree 5 poles (-15.8605, 47.8934) (-15.8626, 47.8965) (-15.8722, 47.9109) (-15.8894, 47.9365) (-15.9143, 47.9733) (-15.947, 48.0213) (-15.9855, 48.0772) (-16.0243, 48.133) (-16.0634, 48.1887) (-16.1029, 48.2442) (-16.1426, 48.2996) (-16.1825, 48.3549) (-16.2228, 48.41) (-16.2633, 48.465) (-16.3041, 48.5199) (-16.3452, 48.5747) (-16.3866, 48.6293) (-16.4282, 48.6838) (-16.47, 48.7381) (-16.5122, 48.7924) (-16.5545, 48.8465) (-16.5972, 48.9004) (-16.64, 48.9543) (-16.6832, 49.008) (-16.7265, 49.0616) (-16.7701, 49.1151) (-16.814, 49.1685) (-16.8581, 49.2217) (-16.9024, 49.2748) (-16.9469, 49.3278) (-16.9917, 49.3807) (-17.0367, 49.4335) (-17.082, 49.4861) (-17.1274, 49.5386) (-17.1731, 49.591) (-17.219, 49.6433) (-17.2651, 49.6954) (-17.3115, 49.7475) (-17.358, 49.7994) (-17.4048, 49.8512) (-17.4518, 49.9029) (-17.499, 49.9544) (-17.5464, 50.0059) (-17.594, 50.0572) (-17.6323, 50.0982) (-17.6611, 50.1289) (-17.6803, 50.1493) (-17.6899, 50.1595) knots 0.396066 0.396066 0.396066 0.396066 0.396066 0.396066 0.4 0.414286 0.428571 0.442857 0.457143 0.471429 0.485714 0.5 0.514286 0.528571 0.542857 0.557143 0.571429 0.585714 0.6 0.614286 0.628571 0.642857 0.657143 0.671429 0.685714 0.7 0.714286 0.728571 0.742857 0.757143 0.771429 0.785714 0.8 0.814286 0.828571 0.842857 0.857143 0.871429 0.885714 0.9 0.914286 0.928571 0.942857 0.957143 0.971429 0.985714 1 1 1 1 1 1
  arc A45 (-17.6899, 50.1595) -> (-18.6906, 49.7953) centre (0, 0) ccw
  spline S90 degree 5 poles (-18.6906, 49.7953) (-18.6914, 49.7813) (-18.6931, 49.7533) (-18.6954, 49.7113) (-18.6984, 49.6553) (-18.7018, 49.5854) (-18.7051, 49.5155) (-18.7081, 49.4456) (-18.7109, 49.3758) (-18.7134, 49.3061) (-18.7157, 49.2364) (-18.7177, 49.1667) (-18.7196, 49.0971) (-18.7211, 49.0276) (-18.7224, 48.9581) (-18.7235, 48.8886) (-18.7243, 48.8192) (-18.7249, 48.7499) (-18.7252, 48.6806) (-18.7253, 48.6114) (-18.7251, 48.5422) (-18.7246, 48.4731) (-18.7239, 48.404) (-18.723, 48.335) (-18.7217, 48.2661) (-18.7202, 48.1972) (-18.7184, 48.1284) (-18.7164, 48.0596) (-18.7141, 47.9909) (-18.7115, 47.9223) (-18.7086, 47.8537) (-18.7055, 47.7853) (-18.702, 47.7169) (-18.6983, 47.6485) (-18.6943, 47.5802) (-18.69, 47.5121) (-18.6854, 47.4439) (-18.6805, 47.3759) (-18.6753, 47.3079) (-18.6698, 47.2401) (-18.664, 47.1723) (-18.6578, 47.1046) (-18.6514, 47.0369) (-18.6456, 46.9792) (-18.641, 46.935) (-18.6377, 46.9043) (-18.6358, 46.8872) (-18.6354, 46.8834) knots -1 -1 -1 -1 -1 -1 -0.985714 -0.971429 -0.957143 -0.942857 -0.928571 -0.914286 -0.9 -0.885714 -0.871429 -0.857143 -0.842857 -0.828571 -0.814286 -0.8 -0.785714 -0.771429 -0.757143 -0.742857 -0.728571 -0.714286 -0.7 -0.685714 -0.671429 -0.657143 -0.642857 -0.628571 -0.614286 -0.6 -0.585714 -0.571429 -0.557143 -0.542857 -0.528571 -0.514286 -0.5 -0.485714 -0.471429 -0.457143 -0.442857 -0.428571 -0.414286 -0.4 -0.396066 -0.396066 -0.396066 -0.396066 -0.396066 -0.396066
  spline S91 degree 3 poles (-18.9434, 46.3663) (-18.8831, 46.391) (-18.8282, 46.4271) (-18.7354, 46.5184) (-18.6984, 46.5727) (-18.6559, 46.6719) (-18.6442, 46.7133) (-18.6316, 46.7979) (-18.6308, 46.8409) (-18.6354, 46.8834) knots 0 0 0 0 0.019532 0.019532 0.039064 0.039064 0.051902 0.051902 0.06474 0.06474 0.06474 0.06474
  arc A46 (-18.9434, 46.3663) -> (-19.391, 46.1809) centre (0, 0) ccw
  spline S92 degree 3 poles (-19.9744, 46.3288) (-19.9336, 46.2781) (-19.8833, 46.2358) (-19.7693, 46.1728) (-19.7067, 46.1528) (-19.5995, 46.1403) (-19.5566, 46.1409) (-19.4718, 46.1529) (-19.4304, 46.1644) (-19.391, 46.1809) knots 0 0 0 0 0.019532 0.019532 0.039064 0.039064 0.051902 0.051902 0.06474 0.06474 0.06474 0.06474
  spline S93 degree 5 poles (-19.9744, 46.3288) (-19.9767, 46.3318) (-19.9875, 46.3452) (-20.0069, 46.3692) (-20.0349, 46.4038) (-20.0716, 46.4487) (-20.1149, 46.501) (-20.1584, 46.5533) (-20.2022, 46.6053) (-20.2463, 46.6572) (-20.2907, 46.7089) (-20.3354, 46.7605) (-20.3803, 46.8119) (-20.4255, 46.8632) (-20.4709, 46.9143) (-20.5166, 46.9652) (-20.5625, 47.016) (-20.6087, 47.0667) (-20.6552, 47.1172) (-20.7019, 47.1676) (-20.7488, 47.2178) (-20.796, 47.2678) (-20.8434, 47.3177) (-20.891, 47.3675) (-20.9389, 47.4171) (-20.987, 47.4666) (-21.0353, 47.5159) (-21.0839, 47.5651) (-21.1327, 47.6142) (-21.1817, 47.6631) (-21.2309, 47.7119) (-21.2803, 47.7605) (-21.33, 47.809) (-21.3798, 47.8574) (-21.4299, 47.9056) (-21.4802, 47.9536) (-21.5307, 48.0016) (-21.5814, 48.0494) (-21.6323, 48.097) (-21.6834, 48.1446) (-21.7347, 48.192) (-21.7862, 48.2392) (-21.8379, 48.2863) (-21.8899, 48.3333) (-21.9315, 48.3708) (-21.9629, 48.3989) (-21.9838, 48.4175) (-21.9943, 48.4269) knots 0.396066 0.396066 0.396066 0.396066 0.396066 0.396066 0.4 0.414286 0.428571 0.442857 0.457143 0.471429 0.485714 0.5 0.514286 0.528571 0.542857 0.557143 0.571429 0.585714 0.6 0.614286 0.628571 0.642857 0.657143 0.671429 0.685714 0.7 0.714286 0.728571 0.742857 0.757143 0.771429 0.785714 0.8 0.814286 0.828571 0.842857 0.857143 0.871429 0.885714 0.9 0.914286 0.928571 0.942857 0.957143 0.971429 0.985714 1 1 1 1 1 1
  arc A47 (-21.9943, 48.4269) -> (-22.9595, 47.9768) centre (0, 0) ccw
  spline S94 degree 5 poles (-22.9595, 47.9768) (-22.959, 47.9628) (-22.9582, 47.9347) (-22.9569, 47.8927) (-22.9549, 47.8367) (-22.9523, 47.7667) (-22.9495, 47.6968) (-22.9464, 47.627) (-22.9431, 47.5572) (-22.9395, 47.4875) (-22.9357, 47.4179) (-22.9317, 47.3483) (-22.9274, 47.2788) (-22.9229, 47.2094) (-22.9182, 47.14) (-22.9132, 47.0707) (-22.908, 47.0015) (-22.9025, 46.9324) (-22.8968, 46.8633) (-22.8908, 46.7944) (-22.8846, 46.7255) (-22.8781, 46.6566) (-22.8714, 46.5879) (-22.8644, 46.5193) (-22.8571, 46.4507) (-22.8496, 46.3822) (-22.8419, 46.3138) (-22.8338, 46.2455) (-22.8255, 46.1773) (-22.817, 46.1091) (-22.8081, 46.0411) (-22.799, 45.9731) (-22.7897, 45.9053) (-22.78, 45.8375) (-22.77, 45.7699) (-22.7598, 45.7023) (-22.7493, 45.6349) (-22.7385, 45.5675) (-22.7274, 45.5003) (-22.716, 45.4331) (-22.7043, 45.3661) (-22.6923, 45.2992) (-22.68, 45.2324) (-22.6692, 45.1754) (-22.6607, 45.1317) (-22.6548, 45.1015) (-22.6514, 45.0845) (-22.6507, 45.0809) knots -1 -1 -1 -1 -1 -1 -0.985714 -0.971429 -0.957143 -0.942857 -0.928571 -0.914286 -0.9 -0.885714 -0.871429 -0.857143 -0.842857 -0.828571 -0.814286 -0.8 -0.785714 -0.771429 -0.757143 -0.742857 -0.728571 -0.714286 -0.7 -0.685714 -0.671429 -0.657143 -0.642857 -0.628571 -0.614286 -0.6 -0.585714 -0.571429 -0.557143 -0.542857 -0.528571 -0.514286 -0.5 -0.485714 -0.471429 -0.457143 -0.442857 -0.428571 -0.414286 -0.4 -0.396066 -0.396066 -0.396066 -0.396066 -0.396066 -0.396066
  spline S95 degree 3 poles (-22.9124, 44.5389) (-22.8545, 44.5687) (-22.803, 44.6095) (-22.7185, 44.7085) (-22.6863, 44.7658) (-22.6527, 44.8684) (-22.6446, 44.9106) (-22.6394, 44.996) (-22.6424, 45.0389) (-22.6507, 45.0809) knots 0 0 0 0 0.019532 0.019532 0.039064 0.039064 0.051902 0.051902 0.06474 0.06474 0.06474 0.06474
  arc A48 (-22.9124, 44.5389) -> (-23.3421, 44.3152) centre (0, 0) ccw
  spline S96 degree 3 poles (-23.9362, 44.4117) (-23.8911, 44.3647) (-23.8373, 44.3269) (-23.7183, 44.2741) (-23.6542, 44.2596) (-23.5464, 44.2566) (-23.5036, 44.2609) (-23.4202, 44.2802) (-23.38, 44.2952) (-23.3421, 44.3152) knots 0 0 0 0 0.019532 0.019532 0.039064 0.039064 0.051902 0.051902 0.06474 0.06474 0.06474 0.06474
  spline S97 degree 5 poles (-23.9362, 44.4117) (-23.9388, 44.4144) (-23.9507, 44.4268) (-23.9721, 44.4491) (-24.003, 44.481) (-24.0435, 44.5226) (-24.0912, 44.571) (-24.1391, 44.6192) (-24.1873, 44.6672) (-24.2357, 44.7151) (-24.2845, 44.7627) (-24.3334, 44.8102) (-24.3827, 44.8575) (-24.4321, 44.9046) (-24.4818, 44.9516) (-24.5318, 44.9984) (-24.582, 45.045) (-24.6324, 45.0914) (-24.6831, 45.1377) (-24.734, 45.1838) (-24.7851, 45.2297) (-24.8365, 45.2755) (-24.8881, 45.3211) (-24.9399, 45.3665) (-24.9919, 45.4118) (-25.0441, 45.4569) (-25.0966, 45.5018) (-25.1492, 45.5466) (-25.2021, 45.5912) (-25.2552, 45.6356) (-25.3084, 45.6799) (-25.3619, 45.7241) (-25.4156, 45.768) (-25.4695, 45.8119) (-25.5236, 45.8555) (-25.5779, 45.899) (-25.6324, 45.9424) (-25.687, 45.9856) (-25.7419, 46.0286) (-25.797, 46.0715) (-25.8522, 46.1143) (-25.9077, 46.1569) (-25.9633, 46.1993) (-26.0191, 46.2416) (-26.0639, 46.2753) (-26.0976, 46.3005) (-26.12, 46.3173) (-26.1313, 46.3256) knots 0.396066 0.396066 0.396066 0.396066 0.396066 0.396066 0.4 0.414286 0.428571 0.442857 0.457143 0.471429 0.485714 0.5 0.514286 0.528571 0.542857 0.557143 0.571429 0.585714 0.6 0.614286 0.628571 0.642857 0.657143 0.671429 0.685714 0.7 0.714286 0.728571 0.742857 0.757143 0.771429 0.785714 0.8 0.814286 0.828571 0.842857 0.857143 0.871429 0.885714 0.9 0.914286 0.928571 0.942857 0.957143 0.971429 0.985714 1 1 1 1 1 1
  arc A49 (-26.1313, 46.3256) -> (-27.0535, 45.7932) centre (0, 0) ccw
  spline S98 degree 5 poles (-27.0535, 45.7932) (-27.0519, 45.7793) (-27.0486, 45.7514) (-27.0436, 45.7096) (-27.0368, 45.654) (-27.0281, 45.5845) (-27.0192, 45.5151) (-27.01, 45.4458) (-27.0006, 45.3766) (-26.991, 45.3075) (-26.9812, 45.2384) (-26.9711, 45.1695) (-26.9608, 45.1006) (-26.9503, 45.0319) (-26.9395, 44.9632) (-26.9285, 44.8946) (-26.9172, 44.8261) (-26.9058, 44.7577) (-26.894, 44.6894) (-26.8821, 44.6212) (-26.8699, 44.5531) (-26.8574, 44.4852) (-26.8447, 44.4173) (-26.8318, 44.3495) (-26.8186, 44.2818) (-26.8052, 44.2142) (-26.7915, 44.1468) (-26.7775, 44.0794) (-26.7633, 44.0122) (-26.7488, 43.945) (-26.7341, 43.878) (-26.7191, 43.8111) (-26.7038, 43.7444) (-26.6883, 43.6777) (-26.6725, 43.6112) (-26.6564, 43.5448) (-26.6401, 43.4785) (-26.6234, 43.4123) (-26.6065, 43.3463) (-26.5893, 43.2804) (-26.5718, 43.2147) (-26.554, 43.149) (-26.5359, 43.0836) (-26.5202, 43.0277) (-26.508, 42.985) (-26.4994, 42.9554) (-26.4946, 42.9388) (-26.4935, 42.9352) knots -1 -1 -1 -1 -1 -1 -0.985714 -0.971429 -0.957143 -0.942857 -0.928571 -0.914286 -0.9 -0.885714 -0.871429 -0.857143 -0.842857 -0.828571 -0.814286 -0.8 -0.785714 -0.771429 -0.757143 -0.742857 -0.728571 -0.714286 -0.7 -0.685714 -0.671429 -0.657143 -0.642857 -0.628571 -0.614286 -0.6 -0.585714 -0.571429 -0.557143 -0.542857 -0.528571 -0.514286 -0.5 -0.485714 -0.471429 -0.457143 -0.442857 -0.428571 -0.414286 -0.4 -0.396066 -0.396066 -0.396066 -0.396066 -0.396066 -0.396066
  spline S99 degree 3 poles (-26.707, 42.3724) (-26.6519, 42.4072) (-26.6042, 42.4523) (-26.5286, 42.5584) (-26.5016, 42.6183) (-26.477, 42.7233) (-26.4727, 42.7661) (-26.475, 42.8516) (-26.4816, 42.8941) (-26.4935, 42.9352) knots 0 0 0 0 0.019532 0.019532 0.039064 0.039064 0.051902 0.051902 0.06474 0.06474 0.06474 0.06474
  arc A50 (-26.707, 42.3724) -> (-27.1156, 42.1121) centre (0, 0) ccw
  spline S100 degree 3 poles (-27.7158, 42.1565) (-27.6669, 42.1136) (-27.61, 42.0807) (-27.4868, 42.0384) (-27.4217, 42.0296) (-27.314, 42.0359) (-27.2717, 42.044) (-27.1904, 42.0705) (-27.1516, 42.089) (-27.1156, 42.1121) knots 0 0 0 0 0.019532 0.019532 0.039064 0.039064 0.051902 0.051902 0.06474 0.06474 0.06474 0.06474
  spline S101 degree 5 poles (-27.7158, 42.1565) (-27.7186, 42.159) (-27.7316, 42.1703) (-27.7549, 42.1906) (-27.7884, 42.2198) (-27.8324, 42.2576) (-27.8841, 42.3017) (-27.9361, 42.3455) (-27.9883, 42.3892) (-28.0407, 42.4326) (-28.0934, 42.4759) (-28.1463, 42.5189) (-28.1995, 42.5617) (-28.2528, 42.6044) (-28.3065, 42.6468) (-28.3603, 42.6891) (-28.4144, 42.7311) (-28.4687, 42.773) (-28.5232, 42.8146) (-28.5779, 42.8561) (-28.6328, 42.8974) (-28.688, 42.9385) (-28.7433, 42.9795) (-28.7989, 43.0202) (-28.8547, 43.0608) (-28.9106, 43.1011) (-28.9668, 43.1413) (-29.0232, 43.1813) (-29.0797, 43.2212) (-29.1365, 43.2608) (-29.1934, 43.3003) (-29.2505, 43.3396) (-29.3079, 43.3788) (-29.3654, 43.4177) (-29.423, 43.4565) (-29.4809, 43.4951) (-29.539, 43.5336) (-29.5972, 43.5718) (-29.6556, 43.6099) (-29.7142, 43.6479) (-29.773, 43.6856) (-29.8319, 43.7232) (-29.891, 43.7606) (-29.9503, 43.7979) (-29.9978, 43.8276) (-30.0336, 43.8498) (-30.0575, 43.8645) (-30.0694, 43.8719) knots 0.396066 0.396066 0.396066 0.396066 0.396066 0.396066 0.4 0.414286 0.428571 0.442857 0.457143 0.471429 0.485714 0.5 0.514286 0.528571 0.542857 0.557143 0.571429 0.585714 0.6 0.614286 0.628571 0.642857 0.657143 0.671429 0.685714 0.7 0.714286 0.728571 0.742857 0.757143 0.771429 0.785714 0.8 0.814286 0.828571 0.842857 0.857143 0.871429 0.885714 0.9 0.914286 0.928571 0.942857 0.957143 0.971429 0.985714 1 1 1 1 1 1
  arc A51 (-30.0694, 43.8719) -> (-30.9417, 43.2611) centre (0, 0) ccw
  spline S102 degree 5 poles (-30.9417, 43.2611) (-30.9389, 43.2473) (-30.9332, 43.2198) (-30.9246, 43.1787) (-30.913, 43.1238) (-30.8982, 43.0554) (-30.8833, 42.987) (-30.8681, 42.9188) (-30.8527, 42.8507) (-30.8371, 42.7826) (-30.8213, 42.7147) (-30.8052, 42.6469) (-30.789, 42.5792) (-30.7725, 42.5116) (-30.7558, 42.4441) (-30.7388, 42.3768) (-30.7217, 42.3095) (-30.7043, 42.2424) (-30.6866, 42.1754) (-30.6688, 42.1085) (-30.6507, 42.0417) (-30.6324, 41.9751) (-30.6138, 41.9086) (-30.595, 41.8422) (-30.576, 41.7759) (-30.5567, 41.7098) (-30.5372, 41.6437) (-30.5174, 41.5779) (-30.4974, 41.5121) (-30.4771, 41.4465) (-30.4566, 41.381) (-30.4358, 41.3157) (-30.4148, 41.2505) (-30.3935, 41.1855) (-30.372, 41.1205) (-30.3502, 41.0558) (-30.3281, 40.9912) (-30.3058, 40.9267) (-30.2831, 40.8624) (-30.2603, 40.7983) (-30.2371, 40.7343) (-30.2136, 40.6705) (-30.1899, 40.6069) (-30.1694, 40.5526) (-30.1535, 40.5111) (-30.1424, 40.4823) (-30.1361, 40.4662) (-30.1348, 40.4627) knots -1 -1 -1 -1 -1 -1 -0.985714 -0.971429 -0.957143 -0.942857 -0.928571 -0.914286 -0.9 -0.885714 -0.871429 -0.857143 -0.842857 -0.828571 -0.814286 -0.8 -0.785714 -0.771429 -0.757143 -0.742857 -0.728571 -0.714286 -0.7 -0.685714 -0.671429 -0.657143 -0.642857 -0.628571 -0.614286 -0.6 -0.585714 -0.571429 -0.557143 -0.542857 -0.528571 -0.514286 -0.5 -0.485714 -0.471429 -0.457143 -0.442857 -0.428571 -0.414286 -0.4 -0.396066 -0.396066 -0.396066 -0.396066 -0.396066 -0.396066
  spline S103 degree 3 poles (-30.2984, 39.8835) (-30.2465, 39.9229) (-30.2029, 39.9721) (-30.1369, 40.0843) (-30.1151, 40.1463) (-30.0998, 40.2531) (-30.0992, 40.2961) (-30.109, 40.3811) (-30.1193, 40.4228) (-30.1348, 40.4627) knots 0 0 0 0 0.019532 0.019532 0.039064 0.039064 0.051902 0.051902 0.06474 0.06474 0.06474 0.06474
  arc A52 (-30.2984, 39.8835) -> (-30.6827, 39.5886) centre (0, 0) ccw
  spline S104 degree 3 poles (-31.2845, 39.5805) (-31.232, 39.542) (-31.1725, 39.5142) (-31.0461, 39.4828) (-30.9804, 39.4797) (-30.8737, 39.4954) (-30.8323, 39.5071) (-30.7536, 39.5406) (-30.7166, 39.5624) (-30.6827, 39.5886) knots 0 0 0 0 0.019532 0.019532 0.039064 0.039064 0.051902 0.051902 0.06474 0.06474 0.06474 0.06474
  spline S105 degree 5 poles (-31.2845, 39.5805) (-31.2876, 39.5827) (-31.3015, 39.5929) (-31.3264, 39.6111) (-31.3624, 39.6372) (-31.4095, 39.6711) (-31.4648, 39.7104) (-31.5204, 39.7496) (-31.5762, 39.7885) (-31.6322, 39.8272) (-31.6885, 39.8657) (-31.745, 39.904) (-31.8016, 39.942) (-31.8586, 39.9799) (-31.9157, 40.0175) (-31.973, 40.0549) (-32.0305, 40.092) (-32.0883, 40.129) (-32.1462, 40.1658) (-32.2043, 40.2023) (-32.2626, 40.2387) (-32.3212, 40.2748) (-32.3799, 40.3108) (-32.4388, 40.3465) (-32.4979, 40.3821) (-32.5571, 40.4174) (-32.6166, 40.4525) (-32.6762, 40.4875) (-32.736, 40.5223) (-32.796, 40.5568) (-32.8562, 40.5912) (-32.9165, 40.6254) (-32.977, 40.6594) (-33.0377, 40.6931) (-33.0986, 40.7268) (-33.1596, 40.7602) (-33.2208, 40.7934) (-33.2821, 40.8265) (-33.3436, 40.8593) (-33.4053, 40.892) (-33.4671, 40.9245) (-33.5291, 40.9568) (-33.5913, 40.9889) (-33.6536, 41.0209) (-33.7035, 41.0463) (-33.7411, 41.0653) (-33.7661, 41.0779) (-33.7787, 41.0842) knots 0.396066 0.396066 0.396066 0.396066 0.396066 0.396066 0.4 0.414286 0.428571 0.442857 0.457143 0.471429 0.485714 0.5 0.514286 0.528571 0.542857 0.557143 0.571429 0.585714 0.6 0.614286 0.628571 0.642857 0.657143 0.671429 0.685714 0.7 0.714286 0.728571 0.742857 0.757143 0.771429 0.785714 0.8 0.814286 0.828571 0.842857 0.857143 0.871429 0.885714 0.9 0.914286 0.928571 0.942857 0.957143 0.971429 0.985714 1 1 1 1 1 1
  arc A53 (-33.7787, 41.0842) -> (-34.5944, 40.3997) centre (0, 0) ccw